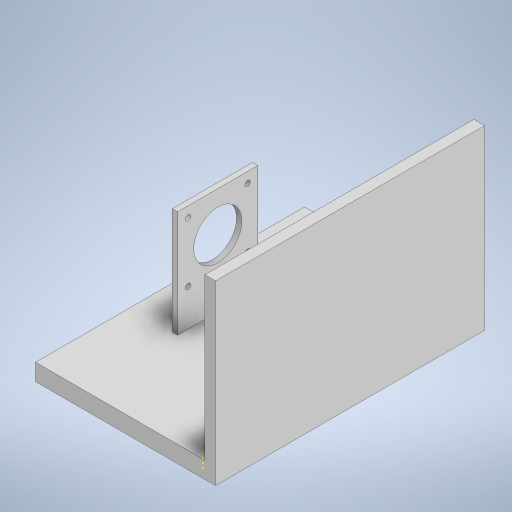
# Autodesk Inventor part: cameraholder
Saved by Autodesk Inventor 2023 (Build 270158000, 158)
## iProperties
Created: 2022-05-04
Part Number: cameraholder
Material: Generic
Document SubType Name: Modeling
Designer: cgbis
Density: 1 g/cm^3
Appearance: Default
Author: cgbis
Autodesk Inventor part; units mm, degrees
(part 1 of 3)
ref_plane "YZ Plane" through (0, 0, 0) normal (1, 0, 0) x (0, 1, 0)
ref_plane "XZ Plane" through (0, 0, 0) normal (0, 1, 0) x (-1, 0, 0)
ref_plane "XY Plane" through (0, 0, 0) normal (0, 0, 1) x (1, 0, 0)
sketch "Sketch1" plane through (0, 0, 0) normal (0, 1, 0) x (-1, 0, 0)
  point P0 (0, 0)
sketch "Sketch2" plane through (0, 0, 0) normal (0, 1, 0) x (-1, 0, 0)
  line L0 (0, 0) -> (85.5, 0)
  line L1 (85.5, 0) -> (85.5, -127.8)
  line L2 (85.5, -127.8) -> (0, -127.8)
  line L3 (0, -127.8) -> (0, 0)
  dimension "d0" = 85.5
  dimension "d1" = 127.8
  constraints: 8 end point, 2 parallel, 1 horizontal, 1 perpendicular
  measures "d0" distance of L1.end L2.end
  measures "d1" distance of L0.end L1.end
extrude "Extrusion1" add sketch "Sketch2" along normal blind 5
sketch "Sketch3" plane through (0, 5, 0) normal (0, 1, 0) x (1, 0, 0)
  line L0 (-85.5, 127.8) -> (-85.5, 0) projected
  line L1 (-85.5, 0) -> (0, 0)
  line L2 (0, 0) -> (0, 127.8)
  line L3 (0, 127.8) -> (-85.5, 127.8)
  line L4 (-85.5, 127.8) -> (-85.5, 0)
  line L5 (-2.4, 2.4) -> (-83.1, 2.4)
  line L6 (-83.1, 2.4) -> (-83.1, 125.4)
  line L7 (-83.1, 125.4) -> (-2.4, 125.4)
  line L8 (-2.4, 125.4) -> (-2.4, 2.4)
  dimension "d6" = 80.7
  dimension "d7" = 123
  constraints: 16 end point, 4 parallel, 2 horizontal, 2 perpendicular
  measures "d6" distance of L6.end L7.end
  measures "d7" distance of L5.end L6.end
extrude "Extrusion2" add sketch "Sketch3" along normal blind 120
sketch "Sketch4" plane through (0, 0, 0) normal (1, 0, 0) x (0, 0, -1)
  line L0 (10, 10) -> (117.8, 10)
  line L1 (117.8, 10) -> (117.8, 115)
  line L2 (117.8, 115) -> (10, 115)
  line L3 (10, 115) -> (10, 10)
  point P0 (0, 0)
  dimension "d10" = 107.8
  dimension "d11" = 105
  constraints: 8 end point, 2 parallel, 1 horizontal, 1 perpendicular
  measures "d10" distance of L2.end L1.end
  measures "d11" distance of L1.end L0.end
extrude "Extrusion3" cut sketch "Sketch4" against normal blind 500
sketch "Sketch5" plane through (0, 0, -127.8) normal (0, 0, -1) x (-1, 0, 0)
  line L0 (10, 10) -> (75.5, 10)
  line L1 (75.5, 10) -> (75.5, 115)
  line L2 (75.5, 115) -> (10, 115)
  line L3 (10, 115) -> (10, 10)
  point P0 (0, 0)
  dimension "d14" = 65.5
  dimension "d15" = 105
  constraints: 8 end point, 2 parallel, 1 horizontal, 1 perpendicular
  measures "d14" distance of L2.end L1.end
  measures "d15" distance of L1.end L0.end
extrude "Extrusion4" cut sketch "Sketch5" against normal blind 500
sketch "Sketch6" plane through (-85.5, 0, -127.8) normal (-1, 0, 0) x (0, 0, 1)
  line L0 (2.4, 125) -> (125.4, 125) projected
  line L1 (63.9, 125) -> (63.9, 0)
  line L2 (0, 0) -> (127.8, 0) projected
  line L3 (63.9, 125) -> (58.9, 125)
  line L4 (58.9, 125) -> (58.9, 0)
  line L5 (58.9, 0) -> (63.9, 0)
  line L6 (63.9, 0) -> (63.9, 125)
  line L7 (63.9, 125) -> (68.9, 125)
  line L8 (68.9, 125) -> (68.9, 0)
  line L9 (68.9, 0) -> (63.9, 0)
  line L10 (63.9, 0) -> (63.9, 125)
  dimension "d18" = 5
  dimension "d19" = 5
  constraints: 18 end point, 4 parallel, 2 horizontal, 2 midpoint, 2 perpendicular, 2 point on line
  measures "d18" distance of L5.end L4.end
  measures "d19" distance of L8.end L9.end
extrude "Extrusion5" add sketch "Sketch6" against normal blind 2.4
sketch "Sketch7" plane through (0, 0, 0) normal (1, 0, 0) x (0, 0, -1)
  line L0 (117.8, 115) -> (10, 115) projected
  line L1 (63.9, 115) -> (63.9, 10)
  line L2 (10, 10) -> (117.8, 10) projected
  line L3 (58.9, 10) -> (58.9, 115) projected
  line L4 (117.8, 10) -> (68.9, 10) projected
  line L5 (58.9, 115) -> (68.9, 115)
  line L6 (68.9, 115) -> (68.9, 10)
  line L7 (68.9, 10) -> (58.9, 10)
  line L8 (58.9, 10) -> (58.9, 115)
  point P0 (0, 0)
  constraints: 10 end point, 2 midpoint, 2 parallel, 1 horizontal, 1 perpendicular
extrude "Extrusion6" add sketch "Sketch7" against normal blind 2.4
sketch "Sketch8" plane through (0, 0, -127.8) normal (0, 0, -1) x (-1, 0, 0)
  line L0 (10, 100) -> (25, 115)
  line L1 (10, 115) -> (75.5, 115) projected
  line L2 (10, 100) -> (31.2132, 100) construction
  line L3 (75.5, 100) -> (60.5, 115)
  line L4 (75.5, 100) -> (96.7132, 100) construction
  line L5 (10, 10) -> (10, 115) projected
  line L6 (10, 25) -> (25, 10)
  line L7 (10, 10) -> (75.5, 10) projected
  line L8 (10, 25) -> (31.2132, 25) construction
  line L9 (75.5, 115) -> (75.5, 10) projected
  line L10 (75.5, 25) -> (60.5, 10)
  line L11 (10, 115) -> (75.5, 115)
  line L12 (75.5, 115) -> (75.5, 10)
  line L13 (75.5, 10) -> (10, 10)
  line L14 (10, 10) -> (10, 115)
  point P0 (0, 0)
  dimension "d24" = 45
  dimension "d25" = 135
  dimension "d26" = 45
  constraints: 22 end point, 6 point on line, 4 horizontal, 3 equal length, 2 parallel, 1 perpendicular
  measures "d24" angle of L2 L0
  measures "d25" angle of L4 L3
  measures "d26" angle of L6 L8
extrude "Extrusion7" add sketch "Sketch8" against normal blind 2.4 contours L5 L1 L0 | L6 L7 L5 | L1 L9 L3 | L10 L9 L7
sketch "Sketch9" plane through (-85.5, 0, 0) normal (0, 0, 1) x (1, 0, 0)
  line L0 (10, 25) -> (10, 100) projected
  line L1 (25, 115) -> (60.5, 115) projected
  line L2 (10, 100) -> (25, 115)
  line L3 (60.5, 115) -> (75.5, 100) projected
  line L4 (25, 115) -> (60.5, 115)
  line L5 (60.5, 115) -> (75.5, 100)
  line L6 (75.5, 100) -> (75.5, 25) projected
  line L7 (75.5, 100) -> (75.5, 25)
  line L8 (75.5, 25) -> (60.5, 10)
  line L9 (25, 10) -> (60.5, 10) projected
  line L10 (10, 25) -> (25, 10) projected
  line L11 (25, 10) -> (10, 25)
  line L12 (10, 25) -> (10, 100)
  line L13 (10, 115) -> (75.5, 115)
  line L14 (75.5, 115) -> (75.5, 10)
  line L15 (75.5, 10) -> (10, 10)
  line L16 (10, 10) -> (10, 115)
  point P0 (85.5, 0)
  point P1 (60.5, 10)
  constraints: 23 end point, 7 equal length, 2 horizontal, 1 perpendicular
extrude "Extrusion8" add sketch "Sketch9" against normal blind 2.4 contours L10 L15 L16 | L16 L13 L2 | L8 L14 L15 | L13 L14 L3
sketch "Sketch10" plane through (0, 0, 0) normal (1, 0, 0) x (0, 0, -1)
  line L0 (10, 115) -> (10, 10) projected
  line L1 (10, 100) -> (25, 115)
  line L2 (58.9, 115) -> (10, 115) projected
  line L3 (10, 100) -> (31.2132, 100) construction
  line L4 (58.9, 10) -> (58.9, 115) projected
  line L5 (58.9, 100) -> (43.9, 115)
  line L6 (58.9, 25) -> (43.9, 10)
  line L7 (10, 10) -> (58.9, 10) projected
  line L8 (10, 25) -> (25, 10)
  line L9 (68.9, 100) -> (83.9, 115)
  line L10 (68.9, 115) -> (117.8, 115) projected
  line L11 (68.9, 100) -> (90.1132, 100) construction
  line L12 (117.8, 115) -> (117.8, 10) projected
  line L13 (117.8, 100) -> (102.8, 115)
  line L14 (117.8, 25) -> (102.8, 10)
  line L15 (117.8, 10) -> (68.9, 10) projected
  line L16 (68.9, 25) -> (83.9, 10)
  line L17 (10, 115) -> (58.9, 115)
  line L18 (58.9, 115) -> (58.9, 10)
  line L19 (58.9, 10) -> (10, 10)
  line L20 (10, 10) -> (10, 115)
  line L21 (68.9, 115) -> (117.8, 115)
  line L22 (117.8, 115) -> (117.8, 10)
  line L23 (117.8, 10) -> (68.9, 10)
  line L24 (68.9, 10) -> (68.9, 115)
  point P0 (0, 0)
  dimension "d31" = 45
  dimension "d32" = 45
  constraints: 36 end point, 11 point on line, 6 perpendicular, 4 horizontal, 4 parallel, 2 equal length
  measures "d31" angle of L3 L1
  measures "d32" angle of L11 L9
extrude "Extrusion9" add sketch "Sketch10" against normal blind 2.4 contours L2 L1 L0 | L8 L7 L0 | L2 L4 L5 | L6 L4 L7 | L24 L10 L9 | L16 L15 L24 | L10 L12 L13 | L14 L12 L15
sketch "Sketch11" plane through (-85.5, 0, -127.8) normal (-1, 0, 0) x (0, 0, 1)
  line L0 (10, 100) -> (25, 115) projected
  line L1 (10, 100) -> (25, 115)
  line L2 (25, 115) -> (43.9, 115) projected
  line L3 (25, 115) -> (43.9, 115)
  line L4 (43.9, 115) -> (58.9, 100)
  line L5 (58.9, 100) -> (58.9, 25)
  line L6 (58.9, 25) -> (43.9, 10) projected
  line L7 (10, 10) -> (58.9, 10) projected
  line L8 (25, 10) -> (10, 25) projected
  line L9 (43.9, 10) -> (25, 10)
  line L10 (25, 10) -> (10, 25)
  line L11 (10, 25) -> (10, 100)
  line L12 (10, 115) -> (10, 10) projected
  line L13 (68.9, 25) -> (68.9, 100) projected
  line L14 (83.9, 115) -> (102.8, 115) projected
  line L15 (68.9, 100) -> (83.9, 115)
  line L16 (83.9, 115) -> (102.8, 115)
  line L17 (102.8, 115) -> (117.8, 100)
  line L18 (117.8, 25) -> (102.8, 10) projected
  line L19 (117.8, 100) -> (117.8, 25)
  line L20 (117.8, 25) -> (102.8, 10)
  line L21 (83.9, 10) -> (102.8, 10) projected
  line L22 (102.8, 10) -> (83.9, 10)
  line L23 (83.9, 10) -> (68.9, 25)
  line L24 (68.9, 25) -> (68.9, 100)
  line L25 (10, 115) -> (58.9, 115)
  line L26 (58.9, 115) -> (58.9, 10)
  line L27 (58.9, 10) -> (10, 10)
  line L28 (10, 10) -> (10, 115)
  line L29 (68.9, 115) -> (117.8, 115)
  line L30 (117.8, 115) -> (117.8, 10)
  line L31 (117.8, 10) -> (68.9, 10)
  line L32 (68.9, 10) -> (68.9, 115)
  point P0 (127.8, 0)
  constraints: 47 end point, 12 equal length, 8 perpendicular, 4 point on line, 2 horizontal
extrude "Extrusion10" add sketch "Sketch11" against normal blind 2.4 contours L12 L25 L0 | L8 L7 L12 | L25 L26 L4 | L6 L26 L7 | L23 L31 L32 | L32 L29 L15 | L18 L30 L31 | L29 L30 L17
sketch "Sketch12" plane through (0, 125, 0) normal (0, 1, 0) x (1, 0, 0)
  line L0 (-83.1, 125.4) -> (-2.4, 125.4) projected
  line L1 (-83.1, 125.4) -> (-83.1, 2.4) projected
  line L2 (-2.4, 125.4) -> (-83.1, 125.4)
  line L3 (-83.1, 125.4) -> (-83.1, 2.4)
  line L4 (-83.1, 2.4) -> (-2.4, 2.4)
  line L5 (-2.4, 2.4) -> (-2.4, 125.4)
  point P0 (0, 0)
  constraints: 8 end point, 2 parallel, 1 horizontal, 1 perpendicular
extrude "Extrusion11" add sketch "Sketch12" against normal blind 4.8
sketch "Sketch13" plane through (0, 125, 0) normal (0, 1, 0) x (1, 0, 0)
  line L0 (-2.4, 2.4) -> (-2.4, 125.4) projected
  line L1 (-83.1, 125.4) -> (-83.1, 2.4) projected
  line L2 (-2.4, 125.4) -> (-83.1, 125.4)
  line L3 (-83.1, 125.4) -> (-83.1, 2.4)
  line L4 (-83.1, 2.4) -> (-2.4, 2.4)
  line L5 (-2.4, 2.4) -> (-2.4, 125.4)
  point P0 (0, 0)
  constraints: 8 end point, 2 parallel, 1 horizontal, 1 perpendicular
extrude "Extrusion12" cut sketch "Sketch13" against normal blind 2.4
sketch "Sketch14" plane through (0, 122.6, 0) normal (0, 1, 0) x (1, 0, 0)
  line L0 (-80.1, 122.4) -> (-5.4, 122.4)
  line L1 (-5.4, 122.4) -> (-5.4, 5.4)
  line L2 (-5.4, 5.4) -> (-80.1, 5.4)
  line L3 (-80.1, 5.4) -> (-80.1, 122.4)
  point P0 (0, 0)
  dimension "d41" = 74.7
  dimension "d42" = 117
  constraints: 8 end point, 2 parallel, 1 horizontal, 1 perpendicular
  measures "d41" distance of L1.end L2.end
  measures "d42" distance of L0.end L1.end
extrude "Extrusion13" cut sketch "Sketch14" against normal blind 10
sketch "Sketch15" plane through (0, 0, 0) normal (1, 0, 0) x (0, 0, -1)
  line L0 (127.8, 0) -> (127.8, 125) projected
  line L1 (0, 125) -> (127.8, 125)
  line L2 (127.8, 125) -> (127.8, 119)
  line L3 (127.8, 119) -> (0, 119)
  line L4 (0, 119) -> (0, 125)
  line L5 (127.8, 125) -> (0, 125) projected
  line L6 (63.9, 125) -> (88.9, 125)
  line L7 (88.9, 125) -> (88.9, 119)
  line L8 (88.9, 119) -> (63.9, 119)
  line L9 (63.9, 119) -> (63.9, 125)
  line L10 (63.9, 125) -> (38.9, 125)
  line L11 (38.9, 125) -> (38.9, 119)
  line L12 (38.9, 119) -> (63.9, 119)
  line L13 (63.9, 119) -> (63.9, 125)
  point P0 (0, 0)
  dimension "d45" = 6
  dimension "d46" = 25
  dimension "d47" = 25
  constraints: 24 end point, 6 parallel, 3 horizontal, 3 perpendicular, 3 point on line, 1 midpoint
  measures "d45" distance of L1.end L2.end
  measures "d46" distance of L7.end L8.end
  measures "d47" distance of L12.end L11.end
extrude "Extrusion14" cut sketch "Sketch15" against normal blind 100 contours L3 L9 L1 L7 | L3 L11 L1 L9
sketch "Sketch16" plane through (0, 0, -127.8) normal (0, 0, -1) x (-1, 0, 0)
  line L0 (0, 125) -> (0, 119) projected
  line L1 (85.5, 0) -> (85.5, 125) projected
  line L2 (0, 125) -> (85.5, 125)
  line L3 (85.5, 125) -> (85.5, 119)
  line L4 (85.5, 119) -> (0, 119)
  line L5 (0, 119) -> (0, 125)
  line L6 (0, 125) -> (85.5, 125) projected
  line L7 (42.75, 125) -> (67.75, 125)
  line L8 (67.75, 125) -> (67.75, 119)
  line L9 (67.75, 119) -> (42.75, 119)
  line L10 (42.75, 119) -> (42.75, 125)
  line L11 (42.75, 125) -> (17.75, 125)
  line L12 (17.75, 125) -> (17.75, 119)
  line L13 (17.75, 119) -> (42.75, 119)
  line L14 (42.75, 119) -> (42.75, 125)
  point P0 (0, 0)
  dimension "d50" = 6
  dimension "d51" = 25
  dimension "d52" = 25
  constraints: 24 end point, 6 parallel, 3 horizontal, 3 perpendicular, 3 point on line, 1 midpoint
  measures "d50" distance of L2.end L3.end
  measures "d51" distance of L8.end L9.end
  measures "d52" distance of L13.end L12.end
extrude "Extrusion15" cut sketch "Sketch16" against normal blind 200 contours L2 L10 L4 L12 | L2 L8 L4 L10
sketch "Sketch17" plane through (-85.5, 0, 0) normal (0, 0, 1) x (1, 0, 0)
  line L0 (17.75, 119) -> (67.75, 119)
  line L1 (67.75, 119) -> (67.75, 118)
  line L2 (67.75, 118) -> (17.75, 118)
  line L3 (17.75, 118) -> (17.75, 119)
  point P0 (85.5, 0)
  dimension "d55" = 1
  constraints: 8 end point, 2 parallel, 1 horizontal, 1 perpendicular
  measures "d55" distance of L0.end L1.end
extrude "Extrusion16" cut sketch "Sketch17" against normal blind 200
sketch "Sketch18" plane through (0, 0, 0) normal (1, 0, 0) x (0, 0, -1)
  line L0 (38.9, 119) -> (38.9, 120.2) projected
  line L1 (38.9, 119) -> (88.9, 119)
  line L2 (88.9, 119) -> (88.9, 118)
  line L3 (88.9, 118) -> (38.9, 118)
  line L4 (38.9, 118) -> (38.9, 119)
  point P0 (0, 0)
  dimension "d58" = 1
  constraints: 8 end point, 2 parallel, 1 horizontal, 1 perpendicular
  measures "d58" distance of L1.end L2.end
extrude "Extrusion17" cut sketch "Sketch18" against normal blind 200
sketch "Sketch19" plane through (0, 0, -127.8) normal (0, 0, -1) x (-1, 0, 0)
  line L0 (17.75, 118) -> (67.75, 118) projected
  line L1 (17.75, 118) -> (67.75, 118)
  line L2 (67.75, 118) -> (67.75, 112)
  line L3 (67.75, 112) -> (17.75, 112)
  line L4 (17.75, 112) -> (17.75, 118)
  point P0 (0, 0)
  dimension "d61" = 50
  dimension "d62" = 6
  constraints: 8 end point, 2 parallel, 1 horizontal, 1 perpendicular
  measures "d61" distance of L2.end L3.end
  measures "d62" distance of L1.end L2.end
extrude "Extrusion18" add sketch "Sketch19" against normal blind 2.4
sketch "Sketch20" plane through (-85.5, 0, -127.8) normal (-1, 0, 0) x (0, 0, 1)
  line L0 (2.4, 118) -> (0, 118) projected
  line L1 (127.8, 100) -> (127.8, 115) projected
  line L2 (0, 118) -> (127.8, 118)
  line L3 (127.8, 118) -> (127.8, 112)
  line L4 (127.8, 112) -> (0, 112)
  line L5 (0, 112) -> (0, 118)
  point P0 (127.8, 0)
  dimension "d65" = 6
  constraints: 8 end point, 2 parallel, 1 horizontal, 1 perpendicular, 1 point on line
  measures "d65" distance of L2.end L3.end
extrude "Extrusion19" add sketch "Sketch20" against normal blind 2.4
sketch "Sketch21" plane through (-85.5, 0, 0) normal (0, 0, 1) x (1, 0, 0)
  line L0 (17.75, 118) -> (67.75, 118) projected
  line L1 (17.75, 118) -> (67.75, 118)
  line L2 (67.75, 118) -> (67.75, 112)
  line L3 (67.75, 112) -> (17.75, 112)
  line L4 (17.75, 112) -> (17.75, 118)
  point P0 (85.5, 0)
  dimension "d68" = 6
  constraints: 8 end point, 2 parallel, 1 horizontal, 1 perpendicular
  measures "d68" distance of L1.end L2.end
extrude "Extrusion20" add sketch "Sketch21" against normal blind 2.4
sketch "Sketch22" plane through (0, 0, 0) normal (1, 0, 0) x (0, 0, -1)
  line L0 (127.8, 0) -> (127.8, 125) projected
  line L1 (0, 118) -> (127.8, 118)
  line L2 (127.8, 118) -> (127.8, 112)
  line L3 (127.8, 112) -> (0, 112)
  line L4 (0, 112) -> (0, 118)
  point P0 (0, 0)
  dimension "d71" = 6
  constraints: 8 end point, 2 parallel, 1 horizontal, 1 perpendicular, 1 point on line
  measures "d71" distance of L1.end L2.end
extrude "Extrusion21" add sketch "Sketch22" against normal blind 2.4
sketch "Sketch23" plane through (0, 125, 0) normal (0, 1, 0) x (1, 0, 0)
  line L0 (-85.5, 127.8) -> (-85.5, 0) projected
  line L1 (-85.5, 127.8) -> (0, 127.8)
  line L2 (0, 127.8) -> (0, 0)
  line L3 (0, 0) -> (-85.5, 0)
  line L4 (-85.5, 0) -> (-85.5, 127.8)
  constraints: 8 end point, 2 parallel, 1 horizontal, 1 perpendicular
extrude "Extrusion22" cut sketch "Sketch23" against normal blind 120
sketch "Sketch24" plane through (0, 5, 0) normal (0, 1, 0) x (1, 0, 0)
  line L0 (0, 127.8) -> (-85.5, 127.8) projected
  line L1 (-42.75, 127.8) -> (-42.75, 0)
  line L2 (-85.5, 0) -> (0, 0) projected
  line L3 (-85.5, 127.8) -> (-85.5, 0) projected
  line L4 (-85.5, 63.9) -> (0, 63.9)
  line L5 (0, 0) -> (0, 127.8) projected
  line L6 (-42.75, 63.9) -> (-36.25, 63.9)
  line L7 (-36.25, 63.9) -> (-36.25, 70.4)
  line L8 (-36.25, 70.4) -> (-42.75, 70.4)
  line L9 (-42.75, 70.4) -> (-42.75, 63.9)
  line L10 (-36.25, 70.4) -> (-49.25, 70.4)
  line L11 (-49.25, 70.4) -> (-49.25, 57.4)
  line L12 (-49.25, 57.4) -> (-36.25, 57.4)
  line L13 (-36.25, 57.4) -> (-36.25, 70.4)
  line L14 (-42.75, 63.9) -> (-34.75, 63.9)
  line L15 (-34.75, 63.9) -> (-34.75, 71.9)
  line L16 (-34.75, 71.9) -> (-42.75, 71.9)
  line L17 (-42.75, 71.9) -> (-42.75, 63.9)
  line L18 (-34.75, 71.9) -> (-50.75, 71.9)
  line L19 (-50.75, 71.9) -> (-50.75, 55.9)
  line L20 (-50.75, 55.9) -> (-34.75, 55.9)
  line L21 (-34.75, 55.9) -> (-34.75, 71.9)
  dimension "d76" = 6.5
  dimension "d77" = 6.5
  dimension "d78" = 13
  dimension "d79" = 13
  dimension "d80" = 8
  dimension "d81" = 8
  dimension "d82" = 16
  dimension "d83" = 16
  constraints: 36 end point, 8 parallel, 5 midpoint, 4 horizontal, 4 perpendicular
  measures "d76" distance of L8.end L7.end
  measures "d77" distance of L7.end L6.end
  measures "d78" distance of L12.end L11.end
  measures "d79" distance of L11.end L10.end
  measures "d80" distance of L16.end L15.end
  measures "d81" distance of L15.end L14.end
  measures "d82" distance of L20.end L19.end
  measures "d83" distance of L19.end L18.end
extrude "Extrusion23" add sketch "Sketch24" along normal blind 25 contours L16 L15 L4 L7 L8 L1 | L1 L10 L11 L4 L19 L18 | L21 L20 L1 L12 L13 L4 | L4 L11 L12 L1 L20 L19
sketch "Sketch25" plane through (0, 5, 0) normal (0, 1, 0) x (1, 0, 0)
  line L0 (-85.5, 0) -> (-85.5, 127.8) projected
  line L1 (-85.5, 127.8) -> (0, 127.8)
  line L2 (0, 127.8) -> (0, 0)
  line L3 (0, 0) -> (-85.5, 0)
  line L4 (-85.5, 0) -> (-85.5, 127.8)
  line L5 (-10, 10) -> (-75.5, 10)
  line L6 (-75.5, 10) -> (-75.5, 117.8)
  line L7 (-75.5, 117.8) -> (-10, 117.8)
  line L8 (-10, 117.8) -> (-10, 10)
  line L9 (-34.75, 71.9) -> (-34.75, 55.9) projected
  line L10 (-34.75, 71.9) -> (-24.75, 71.9)
  line L11 (-24.75, 71.9) -> (-24.75, 81.9)
  line L12 (-24.75, 81.9) -> (-34.75, 81.9)
  line L13 (-34.75, 81.9) -> (-34.75, 71.9)
  line L14 (-50.75, 55.9) -> (-50.75, 71.9) projected
  line L15 (-50.75, 55.9) -> (-60.75, 55.9)
  line L16 (-60.75, 55.9) -> (-60.75, 45.9)
  line L17 (-60.75, 45.9) -> (-50.75, 45.9)
  line L18 (-50.75, 45.9) -> (-50.75, 55.9)
  line L19 (-24.75, 81.9) -> (-60.75, 81.9)
  line L20 (-60.75, 81.9) -> (-60.75, 45.9)
  line L21 (-60.75, 45.9) -> (-24.75, 45.9)
  line L22 (-24.75, 45.9) -> (-24.75, 81.9)
  line L23 (-85.5, 127.8) -> (0, 127.8) projected
  line L24 (-42.75, 127.8) -> (-42.75, 0)
  line L25 (0, 0) -> (-85.5, 0) projected
  line L26 (-85.5, 63.9) -> (0, 63.9)
  line L27 (-42.75, 127.8) -> (-37.75, 127.8)
  line L28 (-37.75, 127.8) -> (-37.75, 81.9)
  line L29 (-37.75, 81.9) -> (-42.75, 81.9)
  line L30 (-42.75, 81.9) -> (-42.75, 127.8)
  line L31 (-42.75, 127.8) -> (-47.75, 127.8)
  line L32 (-47.75, 127.8) -> (-47.75, 81.9)
  line L33 (-47.75, 81.9) -> (-42.75, 81.9)
  line L34 (-42.75, 81.9) -> (-42.75, 127.8)
  line L35 (-85.5, 63.9) -> (-60.75, 63.9)
  line L36 (-60.75, 63.9) -> (-60.75, 68.9)
  line L37 (-60.75, 68.9) -> (-85.5, 68.9)
  line L38 (-85.5, 68.9) -> (-85.5, 63.9)
  line L39 (-60.75, 63.9) -> (-85.5, 63.9)
  line L40 (-85.5, 63.9) -> (-85.5, 58.9)
  line L41 (-85.5, 58.9) -> (-60.75, 58.9)
  line L42 (-60.75, 58.9) -> (-60.75, 63.9)
  line L43 (0, 127.8) -> (0, 0) projected
  line L44 (-85.5, 68.9) -> (0, 68.9)
  line L45 (0, 68.9) -> (0, 58.9)
  line L46 (0, 58.9) -> (-85.5, 58.9)
  line L47 (-85.5, 58.9) -> (-85.5, 68.9)
  line L48 (-47.75, 127.8) -> (-37.75, 127.8)
  line L49 (-37.75, 127.8) -> (-37.75, 0)
  line L50 (-37.75, 0) -> (-47.75, 0)
  line L51 (-47.75, 0) -> (-47.75, 127.8)
  point P0 (-47.75, 10)
  point P1 (-47.75, 45.9)
  point P2 (-75.5, 58.9)
  point P3 (-37.75, 45.9)
  point P4 (-37.75, 10)
  point P5 (-10, 58.9)
  point P6 (-24.75, 58.9)
  point P7 (-37.75, 117.8)
  point P8 (-24.75, 68.9)
  point P9 (-10, 68.9)
  point P10 (-75.5, 68.9)
  point P11 (-47.75, 117.8)
  dimension "d86" = 65.5
  dimension "d87" = 107.8
  dimension "d88" = 10
  dimension "d89" = 10
  dimension "d90" = 10
  dimension "d91" = 10
  dimension "d92" = 5
  dimension "d93" = 5
  dimension "d94" = 5
  dimension "d95" = 5
  constraints: 92 end point, 22 parallel, 11 horizontal, 11 perpendicular, 8 point on line, 4 midpoint
  measures "d86" distance of L6.end L7.end
  measures "d87" distance of L5.end L6.end
  measures "d88" distance of L12.end L11.end
  measures "d89" distance of L11.end L10.end
  measures "d90" distance of L17.end L16.end
  measures "d91" distance of L16.end L15.end
  measures "d92" distance of L28.end L29.end
  measures "d93" distance of L33.end L32.end
  measures "d94" distance of L36.end L35.end
  measures "d95" distance of L40.end L39.end
extrude "Extrusion24" cut sketch "Sketch25" against normal blind 25 contours L41 L20 L16 L17 L21 L51 L5 L6 | L6 L7 L32 L19 L20 L37 | L49 L21 L22 L46 L8 L5 | L7 L8 L44 L22 L11 L12 L19 L28
sketch "Sketch26" plane through (0, 30, 0) normal (0, 1, 0) x (1, 0, 0)
  line L0 (-96.8151, 129.8874) -> (9.0533, 129.8874)
  line L1 (9.0533, 129.8874) -> (9.0533, -6.4667)
  line L2 (9.0533, -6.4667) -> (-96.8151, -6.4667)
  line L3 (-96.8151, -6.4667) -> (-96.8151, 129.8874)
  point P0 (0, 0)
  constraints: 8 end point, 2 parallel, 1 horizontal, 1 perpendicular
extrude "Extrusion25" cut sketch "Sketch26" against normal blind 25
sketch "Sketch27" plane through (0, 5, 0) normal (0, 1, 0) x (1, 0, 0)
  line L0 (0, 127.8) -> (-85.5, 127.8) projected
  line L1 (0, 0) -> (0, 127.8) projected
  line L2 (-85.5, 127.8) -> (0, 127.8)
  line L3 (0, 127.8) -> (0, 0)
  line L4 (0, 0) -> (-85.5, 0)
  line L5 (-85.5, 0) -> (-85.5, 127.8)
  constraints: 8 end point, 2 parallel, 1 horizontal, 1 perpendicular
extrude "Extrusion26" add sketch "Sketch27" against normal blind 5
sketch "Sketch28" plane through (0, 5, 0) normal (0, 1, 0) x (1, 0, 0)
  line L0 (-85.5, 0) -> (-85.5, 127.8) projected
  line L1 (-85.5, 127.8) -> (-70.5, 127.8)
  line L2 (-70.5, 127.8) -> (-70.5, 112.8)
  line L3 (-70.5, 112.8) -> (-85.5, 112.8)
  line L4 (-85.5, 112.8) -> (-85.5, 127.8)
  line L5 (-70.5, 112.8) -> (-65.5, 112.8)
  line L6 (-65.5, 112.8) -> (-65.5, 117.8)
  line L7 (-65.5, 117.8) -> (-70.5, 117.8)
  line L8 (-70.5, 117.8) -> (-70.5, 112.8)
  line L9 (-65.5, 117.8) -> (-75.5, 117.8)
  line L10 (-75.5, 117.8) -> (-75.5, 107.8)
  line L11 (-75.5, 107.8) -> (-65.5, 107.8)
  line L12 (-65.5, 107.8) -> (-65.5, 117.8)
  line L13 (-75.5, 117.8) -> (-65.5, 117.8)
  line L14 (-65.5, 117.8) -> (-65.5, 122.8)
  line L15 (-65.5, 122.8) -> (-75.5, 122.8)
  line L16 (-75.5, 122.8) -> (-75.5, 117.8)
  line L17 (-75.5, 107.8) -> (-65.5, 107.8)
  line L18 (-65.5, 107.8) -> (-65.5, 102.8)
  line L19 (-65.5, 102.8) -> (-75.5, 102.8)
  line L20 (-75.5, 102.8) -> (-75.5, 107.8)
  line L21 (-75.5, 122.8) -> (-75.5, 0)
  line L22 (0, 0) -> (-85.5, 0) projected
  line L23 (-65.5, 122.8) -> (-65.5, 0)
  line L24 (-75.5, 102.8) -> (-65.5, 102.8)
  line L25 (-65.5, 102.8) -> (-65.5, 92.8)
  line L26 (-65.5, 92.8) -> (-75.5, 92.8)
  line L27 (-75.5, 92.8) -> (-75.5, 102.8)
  line L28 (-75.5, 92.8) -> (-65.5, 92.8)
  line L29 (-65.5, 92.8) -> (-65.5, 72.8)
  line L30 (-65.5, 72.8) -> (-75.5, 72.8)
  line L31 (-75.5, 72.8) -> (-75.5, 92.8)
  line L32 (-75.5, 72.8) -> (-65.5, 72.8)
  line L33 (-65.5, 72.8) -> (-65.5, 62.8)
  line L34 (-65.5, 62.8) -> (-75.5, 62.8)
  line L35 (-75.5, 62.8) -> (-75.5, 72.8)
  line L36 (-75.5, 62.8) -> (-65.5, 62.8)
  line L37 (-65.5, 62.8) -> (-65.5, 42.8)
  line L38 (-65.5, 42.8) -> (-75.5, 42.8)
  line L39 (-75.5, 42.8) -> (-75.5, 62.8)
  line L40 (-75.5, 42.8) -> (-65.5, 42.8)
  line L41 (-65.5, 42.8) -> (-65.5, 32.8)
  line L42 (-65.5, 32.8) -> (-75.5, 32.8)
  line L43 (-75.5, 32.8) -> (-75.5, 42.8)
  line L44 (-75.5, 32.8) -> (-65.5, 32.8)
  line L45 (-65.5, 32.8) -> (-65.5, 12.8)
  line L46 (-65.5, 12.8) -> (-75.5, 12.8)
  line L47 (-75.5, 12.8) -> (-75.5, 32.8)
  line L48 (-85.5, 127.8) -> (0, 127.8) projected
  line L49 (-65.5, 0) -> (-45.5, 0)
  line L50 (-45.5, 0) -> (-45.5, 127.8)
  line L51 (-45.5, 127.8) -> (-65.5, 127.8)
  line L52 (-65.5, 127.8) -> (-65.5, 0)
  line L53 (-45.5, 12.8) -> (-35.5, 12.8)
  line L54 (-35.5, 12.8) -> (-35.5, 32.8)
  line L55 (-35.5, 32.8) -> (-45.5, 32.8)
  line L56 (-45.5, 32.8) -> (-45.5, 12.8)
  line L57 (-35.5, 62.8) -> (-45.5, 62.8)
  line L58 (-45.5, 62.8) -> (-45.5, 42.8)
  line L59 (-45.5, 42.8) -> (-35.5, 42.8)
  line L60 (-35.5, 42.8) -> (-35.5, 62.8)
  line L61 (-45.5, 72.8) -> (-35.5, 72.8)
  line L62 (-35.5, 72.8) -> (-35.5, 92.8)
  line L63 (-35.5, 92.8) -> (-45.5, 92.8)
  line L64 (-45.5, 92.8) -> (-45.5, 72.8)
  line L65 (-35.5, 122.8) -> (-45.5, 122.8)
  line L66 (-45.5, 122.8) -> (-45.5, 102.8)
  line L67 (-45.5, 102.8) -> (-35.5, 102.8)
  line L68 (-35.5, 102.8) -> (-35.5, 122.8)
  line L69 (-35.5, 12.8) -> (-15.5, 12.8)
  line L70 (-15.5, 12.8) -> (-15.5, 32.8)
  line L71 (-15.5, 32.8) -> (-35.5, 32.8)
  line L72 (-35.5, 32.8) -> (-35.5, 12.8)
  line L73 (-35.5, 42.8) -> (-15.5, 42.8)
  line L74 (-15.5, 42.8) -> (-15.5, 62.8)
  line L75 (-15.5, 62.8) -> (-35.5, 62.8)
  line L76 (-35.5, 62.8) -> (-35.5, 42.8)
  line L77 (-35.5, 72.8) -> (-15.5, 72.8)
  line L78 (-15.5, 72.8) -> (-15.5, 92.8)
  line L79 (-15.5, 92.8) -> (-35.5, 92.8)
  line L80 (-35.5, 92.8) -> (-35.5, 72.8)
  line L81 (-35.5, 102.8) -> (-15.5, 102.8)
  line L82 (-15.5, 102.8) -> (-15.5, 122.8)
  line L83 (-15.5, 122.8) -> (-35.5, 122.8)
  line L84 (-35.5, 122.8) -> (-35.5, 102.8)
  line L85 (-15.5, 12.8) -> (-5.5, 12.8)
  line L86 (-5.5, 12.8) -> (-5.5, 32.8)
  line L87 (-5.5, 32.8) -> (-15.5, 32.8)
  line L88 (-15.5, 32.8) -> (-15.5, 12.8)
  line L89 (-15.5, 42.8) -> (-5.5, 42.8)
  line L90 (-5.5, 42.8) -> (-5.5, 62.8)
  line L91 (-5.5, 62.8) -> (-15.5, 62.8)
  line L92 (-15.5, 62.8) -> (-15.5, 42.8)
  line L93 (-15.5, 72.8) -> (-5.5, 72.8)
  line L94 (-5.5, 72.8) -> (-5.5, 92.8)
  line L95 (-5.5, 92.8) -> (-15.5, 92.8)
  line L96 (-15.5, 92.8) -> (-15.5, 72.8)
  line L97 (-15.5, 102.8) -> (-5.5, 102.8)
  line L98 (-5.5, 102.8) -> (-5.5, 122.8)
  line L99 (-5.5, 122.8) -> (-15.5, 122.8)
  line L100 (-15.5, 122.8) -> (-15.5, 102.8)
  dimension "d102" = 15
  dimension "d103" = 15
  dimension "d104" = 5
  dimension "d105" = 5
  dimension "d106" = 10
  dimension "d107" = 10
  dimension "d108" = 5
  dimension "d109" = 5
  dimension "d110" = 10
  dimension "d111" = 10
  dimension "d112" = 20
  dimension "d113" = 10
  dimension "d114" = 10
  dimension "d115" = 20
  dimension "d116" = 10
  dimension "d117" = 20
  dimension "d118" = 20
  dimension "d119" = 10
  dimension "d120" = 10
  dimension "d121" = 20
  dimension "d122" = 10
  constraints: 196 end point, 49 parallel, 24 horizontal, 24 perpendicular, 23 point on line, 1 vertical
  measures "d102" distance of L2.end L3.end
  measures "d103" distance of L1.end L2.end
  measures "d104" distance of L7.end L6.end
  measures "d105" distance of L6.end L5.end
  measures "d106" distance of L11.end L10.end
  measures "d107" distance of L10.end L9.end
  measures "d108" distance of L14.end L13.end
  measures "d109" distance of L17.end L18.end
  measures "d110" distance of L24.end L25.end
  measures "d111" distance of L29.end L30.end
  measures "d112" distance of L28.end L29.end
  measures "d113" distance of L33.end L34.end
  measures "d114" distance of L32.end L33.end
  measures "d115" distance of L36.end L37.end
  measures "d116" distance of L40.end L41.end
  measures "d117" distance of L44.end L45.end
  measures "d118" distance of L51.end L50.end
  measures "d119" distance of L55.end L54.end
  measures "d120" distance of L63.end L62.end
  measures "d121" distance of L71.end L70.end
  measures "d122" distance of L87.end L86.end
extrude "Extrusion27" add sketch "Sketch28" along normal blind 10 contours L10 L9 L2 L3 | L3 L5 L12 L11 L10 | L21 L42 L23 L46 | L2 L7 L6 L5 | L16 L15 L2 L9 | L11 L18 L19 L20 | L15 L14 L7 L2 | L21 L34 L23 L38 | L50 L55 L54 L53 | L26 L23 L30 L21 | L65 L68 L67 L50 | L50 L57 L60 L59 | L70 L87 L86 L85 | L63 L62 L61 L50 | L99 L98 L97 L82 | L74 L91 L90 L89 | L95 L94 L93 L78
sketch "Sketch29" plane through (0, 15, 0) normal (0, 1, 0) x (1, 0, 0)
  line L0 (-75.5, 32.8) -> (-75.5, 12.8) projected
  line L1 (-75.5, 22.8) -> (-5.5, 22.8)
  line L2 (-5.5, 12.8) -> (-5.5, 32.8) projected
  line L3 (-75.5, 62.8) -> (-75.5, 42.8) projected
  line L4 (-75.5, 52.8) -> (-5.5, 52.8)
  line L5 (-5.5, 42.8) -> (-5.5, 62.8) projected
  line L6 (-75.5, 72.8) -> (-75.5, 92.8) projected
  line L7 (-75.5, 82.8) -> (-5.5, 82.8)
  line L8 (-5.5, 92.8) -> (-5.5, 72.8) projected
  line L9 (-75.5, 122.8) -> (-75.5, 102.8) projected
  line L10 (-75.5, 112.8) -> (-5.5, 112.8)
  line L11 (-5.5, 122.8) -> (-5.5, 102.8) projected
  line L12 (-75.5, 22.8) -> (-5.5, 22.8)
  line L13 (-5.5, 22.8) -> (-5.5, 30.3)
  line L14 (-5.5, 30.3) -> (-75.5, 30.3)
  line L15 (-75.5, 30.3) -> (-75.5, 22.8)
  line L16 (-75.5, 22.8) -> (-5.5, 22.8)
  line L17 (-5.5, 22.8) -> (-5.5, 15.3)
  line L18 (-5.5, 15.3) -> (-75.5, 15.3)
  line L19 (-75.5, 15.3) -> (-75.5, 22.8)
  line L20 (-75.5, 52.8) -> (-5.5, 52.8)
  line L21 (-5.5, 52.8) -> (-5.5, 45.3)
  line L22 (-5.5, 45.3) -> (-75.5, 45.3)
  line L23 (-75.5, 45.3) -> (-75.5, 52.8)
  line L24 (-75.5, 52.8) -> (-5.5, 52.8)
  line L25 (-5.5, 52.8) -> (-5.5, 60.3)
  line L26 (-5.5, 60.3) -> (-75.5, 60.3)
  line L27 (-75.5, 60.3) -> (-75.5, 52.8)
  line L28 (-75.5, 82.8) -> (-5.5, 82.8)
  line L29 (-5.5, 82.8) -> (-5.5, 75.3)
  line L30 (-5.5, 75.3) -> (-75.5, 75.3)
  line L31 (-75.5, 75.3) -> (-75.5, 82.8)
  line L32 (-5.5, 82.8) -> (-75.5, 82.8)
  line L33 (-75.5, 82.8) -> (-75.5, 90.3)
  line L34 (-75.5, 90.3) -> (-5.5, 90.3)
  line L35 (-5.5, 90.3) -> (-5.5, 82.8)
  line L36 (-75.5, 112.8) -> (-5.5, 112.8)
  line L37 (-5.5, 112.8) -> (-5.5, 105.3)
  line L38 (-5.5, 105.3) -> (-75.5, 105.3)
  line L39 (-75.5, 105.3) -> (-75.5, 112.8)
  line L40 (-75.5, 112.8) -> (-5.5, 112.8)
  line L41 (-5.5, 112.8) -> (-5.5, 120.3)
  line L42 (-5.5, 120.3) -> (-75.5, 120.3)
  line L43 (-75.5, 120.3) -> (-75.5, 112.8)
  line L44 (-75.5, 12.8) -> (-5.5, 12.8)
  line L45 (-5.5, 12.8) -> (-5.5, 15.3)
  line L46 (-5.5, 15.3) -> (-75.5, 15.3)
  line L47 (-75.5, 15.3) -> (-75.5, 12.8)
  line L48 (-75.5, 30.3) -> (-5.5, 30.3)
  line L49 (-5.5, 30.3) -> (-5.5, 32.8)
  line L50 (-5.5, 32.8) -> (-75.5, 32.8)
  line L51 (-75.5, 32.8) -> (-75.5, 30.3)
  line L52 (-75.5, 42.8) -> (-5.5, 42.8)
  line L53 (-5.5, 42.8) -> (-5.5, 45.3)
  line L54 (-5.5, 45.3) -> (-75.5, 45.3)
  line L55 (-75.5, 45.3) -> (-75.5, 42.8)
  line L56 (-5.5, 62.8) -> (-15.5, 62.8) projected
  line L57 (-75.5, 60.3) -> (-5.5, 60.3)
  line L58 (-5.5, 60.3) -> (-5.5, 62.8)
  line L59 (-5.5, 62.8) -> (-75.5, 62.8)
  line L60 (-75.5, 62.8) -> (-75.5, 60.3)
  line L61 (-75.5, 75.3) -> (-5.5, 75.3)
  line L62 (-5.5, 75.3) -> (-5.5, 72.8)
  line L63 (-5.5, 72.8) -> (-75.5, 72.8)
  line L64 (-75.5, 72.8) -> (-75.5, 75.3)
  line L65 (-75.5, 92.8) -> (-5.5, 92.8)
  line L66 (-5.5, 92.8) -> (-5.5, 90.3)
  line L67 (-5.5, 90.3) -> (-75.5, 90.3)
  line L68 (-75.5, 90.3) -> (-75.5, 92.8)
  line L69 (-75.5, 122.8) -> (-5.5, 122.8)
  line L70 (-5.5, 122.8) -> (-5.5, 120.3)
  line L71 (-5.5, 120.3) -> (-75.5, 120.3)
  line L72 (-75.5, 120.3) -> (-75.5, 122.8)
  line L73 (-75.5, 105.3) -> (-5.5, 105.3)
  line L74 (-5.5, 105.3) -> (-5.5, 102.8)
  line L75 (-5.5, 102.8) -> (-75.5, 102.8)
  line L76 (-75.5, 102.8) -> (-75.5, 105.3)
  line L77 (-65.5, 122.8) -> (-65.5, 102.8) projected
  line L78 (-75.5, 12.8) -> (-65.5, 12.8)
  line L79 (-65.5, 12.8) -> (-65.5, 122.8)
  line L80 (-65.5, 122.8) -> (-75.5, 122.8)
  line L81 (-75.5, 122.8) -> (-75.5, 12.8)
  line L82 (-45.5, 122.8) -> (-35.5, 122.8) projected
  line L83 (-35.5, 12.8) -> (-45.5, 12.8) projected
  line L84 (-45.5, 122.8) -> (-35.5, 122.8)
  line L85 (-35.5, 122.8) -> (-35.5, 12.8)
  line L86 (-35.5, 12.8) -> (-45.5, 12.8)
  line L87 (-45.5, 12.8) -> (-45.5, 122.8)
  line L88 (-15.5, 12.8) -> (-5.5, 12.8)
  line L89 (-5.5, 12.8) -> (-5.5, 122.8)
  line L90 (-5.5, 122.8) -> (-15.5, 122.8)
  line L91 (-15.5, 122.8) -> (-15.5, 12.8)
  point P0 (0, 0)
  point P1 (-15.5, 120.3)
  point P2 (-15.5, 105.3)
  point P3 (-15.5, 102.8)
  point P4 (-15.5, 92.8)
  point P5 (-15.5, 90.3)
  point P6 (-15.5, 75.3)
  point P7 (-15.5, 72.8)
  point P8 (-15.5, 60.3)
  point P9 (-15.5, 45.3)
  point P10 (-15.5, 42.8)
  point P11 (-15.5, 32.8)
  point P12 (-15.5, 30.3)
  point P13 (-45.5, 15.3)
  point P14 (-45.5, 32.8)
  point P15 (-45.5, 30.3)
  point P16 (-35.5, 30.3)
  point P17 (-35.5, 32.8)
  point P18 (-45.5, 45.3)
  point P19 (-45.5, 42.8)
  point P20 (-35.5, 42.8)
  point P21 (-35.5, 45.3)
  point P22 (-45.5, 62.8)
  point P23 (-45.5, 60.3)
  point P24 (-35.5, 60.3)
  point P25 (-35.5, 62.8)
  point P26 (-45.5, 75.3)
  point P27 (-45.5, 72.8)
  point P28 (-35.5, 72.8)
  point P29 (-35.5, 75.3)
  point P30 (-45.5, 92.8)
  point P31 (-45.5, 90.3)
  point P32 (-35.5, 90.3)
  point P33 (-35.5, 92.8)
  point P34 (-45.5, 105.3)
  point P35 (-45.5, 102.8)
  point P36 (-35.5, 102.8)
  point P37 (-35.5, 105.3)
  point P38 (-45.5, 120.3)
  point P39 (-35.5, 120.3)
  point P40 (-65.5, 120.3)
  point P41 (-65.5, 105.3)
  point P42 (-65.5, 90.3)
  point P43 (-65.5, 92.8)
  point P44 (-65.5, 72.8)
  point P45 (-65.5, 75.3)
  point P46 (-65.5, 60.3)
  point P47 (-65.5, 62.8)
  point P48 (-65.5, 42.8)
  point P49 (-65.5, 45.3)
  point P50 (-65.5, 30.3)
  point P51 (-65.5, 32.8)
  point P52 (-65.5, 15.3)
  dimension "d125" = 7.5
  dimension "d126" = 7.5
  dimension "d127" = 7.5
  dimension "d128" = 7.5
  dimension "d129" = 7.5
  dimension "d130" = 7.5
  dimension "d131" = 7.5
  dimension "d132" = 7.5
  constraints: 160 end point, 38 parallel, 19 horizontal, 19 perpendicular, 9 point on line, 8 midpoint
  measures "d125" distance of L13.end L12.end
  measures "d126" distance of L16.end L17.end
  measures "d127" distance of L20.end L21.end
  measures "d128" distance of L25.end L24.end
  measures "d129" distance of L28.end L29.end
  measures "d130" distance of L32.end L33.end
  measures "d131" distance of L36.end L37.end
  measures "d132" distance of L41.end L40.end
extrude "Extrusion28" add sketch "Sketch29" along normal blind 2.5 contours L50 L79 L14 L0 | L3 L22 L79 L52 | L50 L85 L14 L87 | L18 L79 L44 L0 | L87 L22 L85 L52 | L50 L2 L14 L91 | L3 L59 L79 L26 | L18 L85 L44 L87 | L91 L22 L5 L52 | L18 L91 L44 L85 | L87 L59 L85 L26 | L6 L30 L79 L63 | L18 L2 L44 L91 | L91 L56 L5 L26 | L87 L30 L85 L63 | L6 L65 L79 L34 | L91 L30 L8 L63 | L87 L65 L85 L34 | L9 L38 L77 L75 | L91 L65 L8 L34 | L87 L38 L85 L75 | L9 L69 L77 L42 | L91 L38 L11 L75 | L87 L69 L85 L42 | L91 L69 L11 L42
sketch "Sketch30" plane through (0, 17.5, 0) normal (0, 1, 0) x (1, 0, 0)
  line L0 (-35.5, 32.8) -> (-35.5, 12.8) projected
  line L1 (-15.5, 15.3) -> (-5.5, 15.3) projected
  line L2 (-35.5, 12.8) -> (-15.5, 12.8)
  line L3 (-15.5, 12.8) -> (-15.5, 15.3)
  line L4 (-15.5, 15.3) -> (-35.5, 15.3)
  line L5 (-35.5, 15.3) -> (-35.5, 12.8)
  point P0 (0, 0)
  constraints: 8 end point, 2 parallel, 1 horizontal, 1 perpendicular
extrude "Extrusion29" cut sketch "Sketch30" against normal blind 2.5
sketch "Sketch31" plane through (-5.5, 5, -12.8) normal (1, 0, 0) x (0, 0, -1)
  line L0 (0, 12.5) -> (2.5, 12.5) projected
  line L1 (2.5, 10) -> (17.5, 10) projected
  line L2 (0, 12.5) -> (2.5, 10)
  line L3 (2.5, 10) -> (17.5, 10)
  line L4 (17.5, 12.5) -> (20, 12.5) projected
  line L5 (17.5, 10) -> (20, 12.5)
  line L6 (0, 0) -> (0, 12.5) projected
  line L7 (0, 12.5) -> (2.5, 12.5)
  line L8 (2.5, 12.5) -> (2.5, 10)
  line L9 (2.5, 10) -> (0, 10)
  line L10 (0, 10) -> (0, 12.5)
  line L11 (20, 0) -> (20, 12.5) projected
  line L12 (17.5, 12.5) -> (20, 12.5)
  line L13 (20, 12.5) -> (20, 10)
  line L14 (20, 10) -> (17.5, 10)
  line L15 (17.5, 10) -> (17.5, 12.5)
  line L16 (30, 12.5) -> (32.5, 12.5) projected
  line L17 (30, 12.5) -> (32.5, 10)
  line L18 (47.5, 10) -> (32.5, 10) projected
  line L19 (32.5, 10) -> (47.5, 10)
  line L20 (50, 0) -> (50, 12.5) projected
  line L21 (47.5, 10) -> (50, 12.5)
  line L22 (30, 12.5) -> (32.5, 12.5)
  line L23 (32.5, 12.5) -> (32.5, 10)
  line L24 (32.5, 10) -> (30, 10)
  line L25 (30, 10) -> (30, 12.5)
  line L26 (47.4746, 12.5) -> (50, 12.5)
  line L27 (50, 12.5) -> (50, 10)
  line L28 (50, 10) -> (47.4746, 10)
  line L29 (47.4746, 10) -> (47.4746, 12.5)
  line L30 (60, 0) -> (60, 12.5) projected
  line L31 (62.5, 10) -> (62.5, 12.5) projected
  line L32 (60, 12.5) -> (62.5, 12.5)
  line L33 (62.5, 12.5) -> (62.5, 10)
  line L34 (62.5, 10) -> (60, 10)
  line L35 (60, 10) -> (60, 12.5)
  line L36 (77.5, 10) -> (77.5, 12.5) projected
  line L37 (80, 0) -> (80, 12.5) projected
  line L38 (77.5, 12.5) -> (80, 12.5)
  line L39 (80, 12.5) -> (80, 10)
  line L40 (80, 10) -> (77.5, 10)
  line L41 (77.5, 10) -> (77.5, 12.5)
  line L42 (60, 12.5) -> (62.5, 10)
  line L43 (80, 12.5) -> (77.5, 10)
  line L44 (92.5, 10) -> (107.5, 10) projected
  line L45 (90.0061, 12.4939) -> (92.5, 10)
  line L46 (110, 0) -> (110, 12.5) projected
  line L47 (110, 12.5) -> (107.5, 10)
  line L48 (90, 12.5) -> (92.5, 12.5)
  line L49 (92.5, 12.5) -> (92.5, 10)
  line L50 (92.5, 10) -> (90, 10)
  line L51 (90, 10) -> (90, 12.5)
  line L52 (110, 12.5) -> (107.5, 12.5)
  line L53 (107.5, 12.5) -> (107.5, 10)
  line L54 (107.5, 10) -> (110, 10)
  line L55 (110, 10) -> (110, 12.5)
  point P0 (-12.8, -5)
  constraints: 84 end point, 18 equal length, 12 perpendicular, 10 point on line, 8 horizontal
extrude "Extrusion30" cut sketch "Sketch31" against normal blind 300 contours L0 L8 L2 | L4 L5 L15 | L16 L23 L17 | L18 L29 L26 L21 | L32 L31 L42 | L36 L38 L43 | L47 L53 L52
sketch "Sketch32" plane through (-5.5, 5, -102.8) normal (1, 0, 0) x (0, 0, -1)
  line L0 (0, 0) -> (0, 12.5) projected
  line L1 (0, 12.5) -> (2.5, 12.5)
  line L2 (2.5, 12.5) -> (2.5, 10)
  line L3 (2.5, 10) -> (0, 10)
  line L4 (0, 10) -> (0, 12.5)
  line L5 (0, 12.5) -> (2.5, 12.5) projected
  line L6 (0, 12.5) -> (2.5, 10)
  point P0 (-102.8, -5)
  constraints: 10 end point, 2 parallel, 1 horizontal, 1 perpendicular
extrude "Extrusion31" cut sketch "Sketch32" against normal blind 300 contours L1 L2 L6
sketch "Sketch33" plane through (0, 5, 0) normal (0, 1, 0) x (1, 0, 0)
  line L0 (-75.5, 122.8) -> (-65.5, 122.8) projected
  line L1 (-75.5, 122.8) -> (0, 122.8)
  line L2 (0, 122.8) -> (0, 131.7)
  line L3 (0, 131.7) -> (-75.5, 131.7)
  line L4 (-75.5, 131.7) -> (-75.5, 122.8)
  line L5 (-85.5, 0) -> (-85.5, 127.8) projected
  line L6 (-75.5, 131.7) -> (-85.5, 131.7)
  line L7 (-85.5, 131.7) -> (-85.5, 122.8)
  line L8 (-85.5, 122.8) -> (-75.5, 122.8)
  line L9 (-75.5, 122.8) -> (-75.5, 131.7)
  point P0 (0, 0)
  dimension "d141" = 8.9
  constraints: 16 end point, 4 parallel, 2 horizontal, 2 perpendicular, 2 point on line
  measures "d141" distance of L2.end L1.end
extrude "Extrusion32" add sketch "Sketch33" against normal blind 5
sketch "Sketch34" plane through (0, 5, 0) normal (0, 1, 0) x (1, 0, 0)
  line L0 (-75.5, 12.8) -> (-75.5, 32.8) projected
  line L1 (0, 131.7) -> (0, 0) projected
  line L2 (-75.5, 12.8) -> (0, 12.8)
  line L3 (0, 12.8) -> (0, 3.9)
  line L4 (0, 3.9) -> (-75.5, 3.9)
  line L5 (-75.5, 3.9) -> (-75.5, 12.8)
  line L6 (0, 3.9) -> (-85.5328, 3.9)
  line L7 (-85.5328, 3.9) -> (-85.5328, 0)
  line L8 (-85.5328, 0) -> (0, 0)
  line L9 (0, 0) -> (0, 3.9)
  dimension "d144" = 8.9
  constraints: 16 end point, 4 parallel, 2 horizontal, 2 perpendicular, 1 point on line
  measures "d144" distance of L2.end L3.end
extrude "Extrusion33" cut sketch "Sketch34" against normal blind 5 contours L1 L8 L7 L6 L4
sketch "Sketch35" plane through (0, 5, 0) normal (0, 1, 0) x (1, 0, 0)
  line L0 (-75.5, 12.8) -> (-75.5, 32.8) projected
  line L1 (-85.5, 131.7) -> (0, 131.7) projected
  line L2 (-75.5, 12.8) -> (-83.25, 12.8)
  line L3 (-83.25, 12.8) -> (-83.25, 131.7)
  line L4 (-83.25, 131.7) -> (-75.5, 131.7)
  line L5 (-75.5, 131.7) -> (-75.5, 12.8)
  line L6 (-85.5, 3.9) -> (-85.5, 131.7) projected
  line L7 (-83.25, 131.7) -> (-85.5, 131.7)
  line L8 (-85.5, 131.7) -> (-85.5, 3.9)
  line L9 (-85.5, 3.9) -> (-83.25, 3.9)
  line L10 (-83.25, 3.9) -> (-83.25, 131.7)
  point P0 (0, 0)
  dimension "d147" = 7.75
  constraints: 16 end point, 4 parallel, 2 horizontal, 2 perpendicular, 1 point on line
  measures "d147" distance of L3.end L4.end
extrude "Extrusion34" cut sketch "Sketch35" against normal blind 5 contours L10 L9 L6 L1 L3
sketch "Sketch36" plane through (0, 5, 0) normal (0, 1, 0) x (1, 0, 0)
  line L0 (-5.5, 32.8) -> (-5.5, 12.8) projected
  line L1 (-5.5, 12.8) -> (2.25, 12.8)
  line L2 (2.25, 12.8) -> (2.25, 131.7)
  line L3 (2.25, 131.7) -> (-5.5, 131.7)
  line L4 (-5.5, 131.7) -> (-5.5, 12.8)
  line L5 (-5.5, 12.8) -> (2.25, 12.8)
  line L6 (2.25, 12.8) -> (2.25, 3.9)
  line L7 (2.25, 3.9) -> (-5.5, 3.9)
  line L8 (-5.5, 3.9) -> (-5.5, 12.8)
  point P0 (0, 0)
  dimension "d150" = 7.75
  constraints: 16 end point, 4 parallel, 2 horizontal, 2 perpendicular, 1 point on line
  measures "d150" distance of L3.end L2.end
extrude "Extrusion35" add sketch "Sketch36" against normal blind 5
sketch "Sketch37" plane through (0, 15, 0) normal (0, 1, 0) x (1, 0, 0)
  line L0 (-116.9368, 146.7159) -> (75.9783, 146.7159)
  line L1 (75.9783, 146.7159) -> (75.9783, -62.9122)
  line L2 (75.9783, -62.9122) -> (-116.9368, -62.9122)
  line L3 (-116.9368, -62.9122) -> (-116.9368, 146.7159)
  point P0 (0, 0)
  constraints: 8 end point, 2 parallel, 1 horizontal, 1 perpendicular
extrude "Extrusion36" cut sketch "Sketch37" along normal blind 10
sketch "Sketch38" plane through (0, 15, 0) normal (0, 1, 0) x (1, 0, 0)
  line L0 (-75.5, 102.8) -> (-75.5, 122.8) projected
  line L1 (-75.5, 112.8) -> (-5.5, 112.8)
  line L2 (-5.5, 102.8) -> (-5.5, 122.8) projected
  line L3 (-75.5, 72.8) -> (-75.5, 92.8) projected
  line L4 (-75.5, 82.8) -> (-5.5, 82.8)
  line L5 (-5.5, 72.8) -> (-5.5, 92.8) projected
  line L6 (-5.5, 42.8) -> (-5.5, 62.8) projected
  line L7 (-5.5, 52.8) -> (-75.5, 52.8)
  line L8 (-75.5, 32.8) -> (-75.5, 12.8) projected
  line L9 (-75.5, 22.8) -> (-5.5, 22.8)
  line L10 (-5.5, 32.8) -> (-5.5, 12.8) projected
  line L11 (-65.5, 102.8) -> (-65.5, 122.8) projected
  line L12 (-65.5, 112.8) -> (-75.5, 112.8)
  line L13 (-70.5, 112.8) -> (-70.5, 123.8)
  line L14 (-70.5, 123.8) -> (-70.5, 101.8)
  line L15 (-70.5, 101.8) -> (-59.5, 112.8)
  line L16 (-59.5, 112.8) -> (-70.5, 123.8)
  line L17 (-70.5, 123.8) -> (-81.5, 112.8)
  line L18 (-81.5, 112.8) -> (-70.5, 101.8)
  line L19 (-75.5, 122.8) -> (-65.5, 122.8) projected
  line L20 (-75.5, 122.8) -> (-65, 122.8)
  line L21 (-65, 122.8) -> (-65, 102.8)
  line L22 (-65, 102.8) -> (-75.5, 102.8)
  line L23 (-75.5, 102.8) -> (-75.5, 122.8)
  point P0 (0, 0)
  point P1 (-71.5, 102.8)
  point P2 (-75.5, 106.8)
  point P3 (-69.5, 102.8)
  point P4 (-65.5, 106.8)
  point P5 (-69.5, 122.8)
  point P6 (-65.5, 118.8)
  point P7 (-71.5, 122.8)
  point P8 (-75.5, 118.8)
  dimension "d155" = 11
  dimension "d156" = 22
  dimension "d157" = 45
  constraints: 30 end point, 9 midpoint, 4 perpendicular, 3 point on line, 2 horizontal, 2 parallel, 1 collinear, 1 vertical
  measures "d155" distance of L13.start L13.end
  measures "d156" distance of L13.end L14.end
  measures "d157" angle of L15 L14
extrude "Extrusion37" add sketch "Sketch38" along normal blind 3 contours L0 L18 L22 | L0 L19 L17 | L15 L11 L22 | L16 L19 L11
chamfer "Chamfer1" distance 2.5 distance2 3 1 edges at (-73.5, 18, -120.8) measured on face at (-73.8536, 18, -121.1536)
chamfer "Chamfer2" distance 2.5 distance2 3 1 edges at (-67.5, 18, -120.8) measured on face at (-67.1464, 18, -121.1536)
chamfer "Chamfer3" distance 2.5 distance2 3 1 edges at (-73.5, 18, -104.8) measured on face at (-73.8536, 18, -104.4464)
chamfer "Chamfer4" distance 2.5 distance2 3 1 edges at (-67.5, 18, -104.8) measured on face at (-67.1464, 18, -104.4464)
sketch "Sketch39" plane through (0, 15, 0) normal (0, 1, 0) x (1, 0, 0)
  point P0 (0, 0)
sketch "Sketch40" plane through (0, 15, 0) normal (0, 1, 0) x (1, 0, 0)
  line L0 (-45.5, 102.8) -> (-45.5, 122.8) projected
  line L1 (-45.5, 112.8) -> (-35.5, 112.8)
  line L2 (-35.5, 122.8) -> (-35.5, 102.8) projected
  line L3 (-40.5, 112.8) -> (-40.5, 123.8)
  line L4 (-40.5, 123.8) -> (-29.5, 112.8)
  line L5 (-29.5, 112.8) -> (-40.5, 101.8)
  line L6 (-40.5, 101.8) -> (-51.5, 112.8)
  line L7 (-51.5, 112.8) -> (-40.5, 123.8)
  line L8 (-45.5, 122.8) -> (-35.5, 122.8)
  line L9 (-35.5, 122.8) -> (-35.5, 102.8)
  line L10 (-35.5, 102.8) -> (-45.5, 102.8)
  line L11 (-45.5, 102.8) -> (-45.5, 122.8)
  point P0 (0, 0)
  point P1 (-41.5, 102.8)
  point P2 (-45.5, 106.8)
  point P3 (-39.5, 102.8)
  point P4 (-35.5, 106.8)
  point P5 (-39.5, 122.8)
  point P6 (-35.5, 118.8)
  point P7 (-41.5, 122.8)
  point P8 (-45.5, 118.8)
  dimension "d172" = 11
  dimension "d173" = 45
  dimension "d174" = 90
  constraints: 20 end point, 3 midpoint, 2 parallel, 2 perpendicular, 2 point on line, 1 horizontal, 1 vertical
  measures "d172" distance of L3.start L3.end
  measures "d173" angle of L3 L4
  measures "d174" angle of L4 L5
extrude "Extrusion38" add sketch "Sketch40" along normal blind 3 contours L0 L6 L10 | L5 L2 L10 | L0 L8 L7 | L4 L8 L2
chamfer "Chamfer5" distance 2.5 distance2 3 1 edges at (-43.5, 18, -120.8) measured on face at (-43.8536, 18, -121.1536)
chamfer "Chamfer6" distance 2.5 distance2 3 1 edges at (-37.5, 18, -120.8) measured on face at (-37.1464, 18, -121.1536)
chamfer "Chamfer7" distance 2.5 distance2 3 1 edges at (-43.5, 18, -104.8) measured on face at (-43.8536, 18, -104.4464)
chamfer "Chamfer8" distance 2.5 distance2 3 1 edges at (-37.5, 18, -104.8) measured on face at (-37.1464, 18, -104.4464)